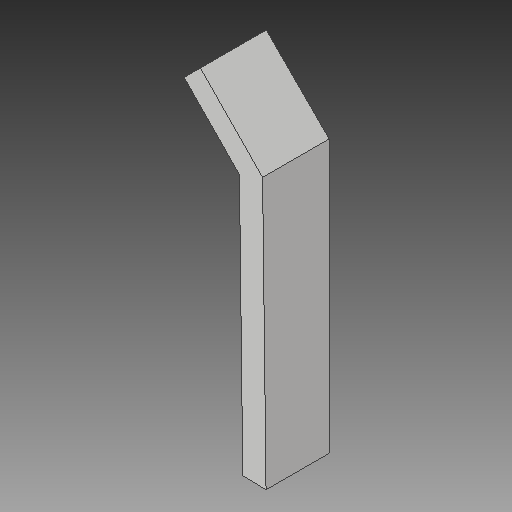
# Autodesk Inventor part: frame3
Saved by Autodesk Inventor 2019 (Build 230136000, 136)
## iProperties
Created: 2020-03-15
Part Number: frame3
Material: Generic
Document SubType Name: Modeling
Designer: Pulag
Density: 1 g/cm^3
Appearance: Default
Author: Pulag
Autodesk Inventor part; units mm, degrees
ref_plane "YZ Plane" through (0, 0, 0) normal (1, 0, 0) x (0, 1, 0)
ref_plane "XZ Plane" through (0, 0, 0) normal (0, 1, 0) x (-1, 0, 0)
ref_plane "XY Plane" through (0, 0, 0) normal (0, 0, 1) x (1, 0, 0)
sketch "Sketch1" plane through (0, 0, 0) normal (0, 0, 1) x (1, 0, 0)
  line L0 (-49.6667, 14.3759) -> (-49.6743, 36.8741) projected
  line L1 (-34.4709, 14.3764) -> (-49.6667, 14.3759) projected
  line L2 (-34.4709, 14.3764) -> (-34.4693, 9.5768) projected
  line L3 (-31.97, 9.5769) -> (-34.4693, 9.5768) projected
  line L4 (-31.97, 9.5769) -> (-31.9716, 14.3765) projected
  line L5 (-31.9716, 14.3765) -> (-27.4729, 14.3767) projected
  line L6 (-27.4729, 14.3767) -> (-27.4804, 36.8749) projected
  line L7 (-31.9792, 36.8747) -> (-27.4804, 36.8749) projected
  line L8 (-31.9792, 36.8747) -> (-31.9808, 41.6744) projected
  line L9 (-34.4801, 41.6743) -> (-31.9808, 41.6744) projected
  line L10 (-34.4785, 36.8746) -> (-34.4801, 41.6743) projected
  line L11 (-34.4785, 36.8746) -> (-49.6743, 36.8741) projected
  line L12 (-13.1949, 46.2616) -> (36.8051, 46.2616) construction
  line L13 (-39.4709, 69.4116) -> (-51.2007, 81.1414)
  line L14 (-51.2007, 81.1414) -> (-47.6652, 84.6769)
  line L15 (-47.6652, 84.6769) -> (-34.4709, 71.4827)
  line L16 (-34.4709, 14.3764) -> (-39.4709, 14.3764)
  line L17 (-39.4709, 14.3764) -> (-39.4709, 69.4116)
  line L18 (-34.4709, 64.4116) -> (-34.4709, 14.3764)
  line L19 (-34.4709, 64.4116) -> (-34.4709, 71.4827)
  point P0 (0, 0)
  dimension "d2" = 5
  constraints: 16 end point, 2 horizontal, 2 parallel, 2 perpendicular, 1 point on line, 1 other
  measures "d2" distance of L13.end L14.end
ref_plane "Work Plane1" through (-48.7843, 8.2823, 12.8261) normal (-0.0234916, -0.0126579, 0.9996439) x (0.999724, -0.0003364, 0.0234893)
extrude "Extrusion1" add sketch "Sketch1" along normal up to surface contours L17 L11 L10 L9 L18 L1 | L17 L13 L14 L15 L19 L18 L9 L10 L11 surface through (-48.7843, 8.2823, 12.8261) normal (-0.0234916, -0.0126579, 0.9996439)
body "Solid1"
